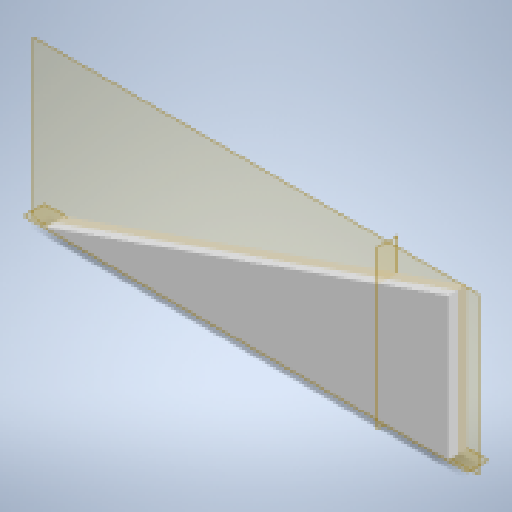
# Autodesk Inventor part: Ребро жётскости крыла
Saved by Autodesk Inventor 2023.2 (Build 272271030, 271C)
## iProperties
Created: 2024-03-20
Part Number: Ребро жётскости крыла
Material: Типовые
Document SubType Name: Modeling
Designer: I9232
Density: 1 g/cm^3
Appearance: По умолчанию
Author: I9232
Autodesk Inventor part; units mm, degrees
sketch "Эскиз1" plane through (0, 0, 0) normal (0, 0, 1) x (1, 0, 0)
  line L0 (-70.2411, 0) -> (14.7589, 0)
  line L1 (14.7589, 0) -> (14.7589, 30)
  line L2 (14.7589, 30) -> (-70.2411, 0)
  point P0 (0, 0)
  dimension "d0" = 30
  dimension "d1" = 85
  constraints: 6 end point, 1 horizontal, 1 perpendicular
  measures "d0" distance of L0.end L1.end
  measures "d1" distance of L0.start L0.end
extrude "Выдавливание1" add sketch "Эскиз1" along normal mid plane 4
